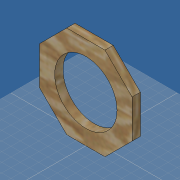
# Autodesk Inventor part: Korpus_Motor_18mm
Saved by Autodesk Inventor 2019 (Build 230136000, 136)
## iProperties
Created: 2020-08-02
Part Number: Korpus_Motor_18mm
Material: Generisch
Document SubType Name: Modeling
Designer: Stefan
Mass: 338.818 g
Surface Area: 572.098 cm^2
Volume: 338.818 cm^3
Density: 1 g/cm^3
Appearance: Sperrholz - verwittert
Author: Stefan
Autodesk Inventor part; units mm, degrees
ref_plane "YZ Plane" through (0, 0, 0) normal (1, 0, 0) x (0, 1, 0)
ref_plane "XZ Plane" through (0, 0, 0) normal (0, 1, 0) x (-1, 0, 0)
ref_plane "XY Plane" through (0, 0, 0) normal (0, 0, 1) x (1, 0, 0)
sketch "Skizze2" plane through (0, 0, 0) normal (0, 0, 1) x (1, 0, 0)
  circle A0 centre (0, 0) radius 67.5
  line L0 (-41.4214, 100) -> (41.4214, 100)
  line L1 (41.4214, 100) -> (100, 41.4214)
  line L2 (100, 41.4214) -> (100, -41.4214)
  line L3 (100, -41.4214) -> (41.4214, -100)
  line L4 (41.4214, -100) -> (-41.4214, -100)
  line L5 (-41.4214, -100) -> (-100, -41.4214)
  line L6 (-100, -41.4214) -> (-100, 41.4214)
  line L7 (-100, 41.4214) -> (-41.4214, 100)
  dimension "d7" = 135
  dimension "d11" = 200
  constraints: 16 end point, 4 coincident, 1 centre point, 1 horizontal, 17 other
  measures "d7" diameter of A0
  measures "d11" distance between parallel lines of L4 L0
extrude "Extrusion2" add sketch "Skizze2" along normal blind 18
equation "\"kg_thickness\" = 4.9"
equation "\"ht_thickness\" = 1.9"
equation "\"case_thickness\" = 18"
equation "\"inner_thickness\" = 15"
equation "\"gap_fit\" = 0.1"
equation "\"gap_slide\" = 0.2"
equation "\"gap_air\" = 1"
equation "\"bore_diameter\" = 73"
equation "\"mdf_thickness\" = 6"
equation "\"tape_width\" = 15"
equation "\"tape_thickness\" = 3"
equation "\"inner_depth\" = 255"
